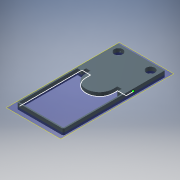
# Autodesk Inventor part: Cup_Dispenser_Slider
Saved by Autodesk Inventor 2016 (Build 200138000, 138)
## iProperties
Created: 2015-07-09
Part Number: Cup_Dispenser_Slider
Material: Generic
Document SubType Name: Modeling
Designer: marku
Density: 1 g/cm^3
Appearance: Lead
Author: marku
Autodesk Inventor part; units mm, degrees
ref_plane "YZ Plane" through (0, 0, 0) normal (1, 0, 0) x (0, 1, 0)
ref_plane "XZ Plane" through (0, 0, 0) normal (0, 1, 0) x (-1, 0, 0)
ref_plane "XY Plane" through (0, 0, 0) normal (0, 0, 1) x (1, 0, 0)
sketch "Sketch2" plane through (0, 0, 0) normal (0, 0, 1) x (1, 0, 0)
  line L0 (54, 117.2078) -> (54, -112.7922)
  arc A0 (50, -116.7922) -> (54, -112.7922) centre (50, -112.7922) ccw
  line L1 (50, -116.7922) -> (-50, -116.7922)
  arc A1 (-54, -112.7922) -> (-50, -116.7922) centre (-50, -112.7922) ccw
  line L2 (-54, -112.7922) -> (-54, 117.2078)
  line L3 (51, 117.2078) -> (51, -112.7922)
  arc A2 (50, -113.7922) -> (51, -112.7922) centre (50, -112.7922) ccw
  line L4 (50, -113.7922) -> (-50, -113.7922)
  arc A3 (-51, -112.7922) -> (-50, -113.7922) centre (-50, -112.7922) ccw
  line L5 (-51, -112.7922) -> (-51, 117.2078)
  line L6 (54, 117.2078) -> (-54, 117.2078)
  line L7 (-51, 114.2078) -> (51, 114.2078)
  dimension "d99" = 3
  dimension "d100" = 3
  constraints: 16 end point, 8 point on circle, 4 centre point, 2 horizontal, 2 point on line, 2 vertical, 1 perpendicular, 14 other
  measures "d99" distance between parallel lines of L0 L3
  measures "d100" distance between parallel lines of L6 L7
ref_plane "Work Plane1" through (-57, -119.7922, 15) normal (0, 0, -1) x (0, 1, 0)
ref_plane "Work Plane3" through (-57, -119.7922, 15) normal (0, 0, -1) x (0, 1, 0)
extrude "Extrusion1" add sketch "Sketch2" along normal up to surface (15 mm away) contours L0 A0 L1 A1 L2 L6 L5 A3 L4 A2 L3 | L3 L7 L5 L6
sketch "Sketch3" plane through (0, 0, 0) normal (0, 0, -1) x (-1, 0, 0)
  arc A0 (31.25, 57.2078) -> (-31.25, 57.2078) centre (0, 57.2078) ccw
  line L0 (-54, -112.7922) -> (-54, 114.2078) projected
  line L1 (-31.25, 57.2078) -> (-31.25, 47.2078)
  line L2 (-31.25, 47.2078) -> (-51, 47.2078)
  line L3 (31.25, 57.2078) -> (31.25, 47.2078)
  line L4 (31.25, 47.2078) -> (51, 47.2078)
  line L5 (-51, 114.2078) -> (51, 114.2078) projected
  line L6 (-51, -112.7922) -> (-51, 114.2078) projected
  line L7 (51, 114.2078) -> (51, -112.7922) projected
  circle A1 centre (0, 57.2078) radius 54 construction
  point P0 (0, 0)
  dimension "d8" = 31.25
  dimension "d9" = 10
  dimension "d10" = 10
  constraints: 8 end point, 4 point on line, 2 perpendicular, 2 point on circle, 1 centre point, 1 coincident, 1 tangent, 1 vertical
  measures "d8" radius of A0
  measures "d9" distance of L1.start L1.end
  measures "d10" distance of L3.start L3.end
extrude "Extrusion2" add sketch "Sketch3" against normal blind 3
ref_plane "Work Plane2" through (0, 0, 6) normal (0, 0, -1) x (-1, 0, 0)
sketch "Sketch4" plane through (0, 0, 6) normal (0, 0, -1) x (-1, 0, 0)
  line L0 (-31.25, 47.2078) -> (-51, 47.2078) construction
  circle A0 centre (0, 20.6666) radius 41 construction
  arc A1 (-31.25, 20.6666) -> (31.25, 20.6666) centre (0, 20.6666) ccw
  line L1 (-31.25, 20.6666) -> (-31.25, 30.6666)
  line L2 (31.25, 20.6666) -> (31.25, 30.6666)
  line L3 (31.25, 30.6666) -> (51, 30.6666)
  line L4 (-31.25, 30.6666) -> (-51, 30.6666)
  arc A2 (-51, -112.7922) -> (-50, -113.7922) centre (-50, -112.7922) ccw projected
  line L5 (-50, -113.7922) -> (50, -113.7922) projected
  arc A3 (50, -113.7922) -> (51, -112.7922) centre (50, -112.7922) ccw projected
  line L6 (51, -112.7922) -> (51, 114.2078) projected
  line L7 (51, 114.2078) -> (-51, 114.2078) projected
  line L8 (-51, 114.2078) -> (-51, -112.7922) projected
  arc A4 (-54, -112.7922) -> (-50, -116.7922) centre (-50, -112.7922) ccw projected
  line L9 (-54, -112.7922) -> (-54, 117.2078) projected
  line L10 (-54, 117.2078) -> (54, 117.2078) projected
  line L11 (54, 117.2078) -> (54, -112.7922) projected
  arc A5 (50, -116.7922) -> (54, -112.7922) centre (50, -112.7922) ccw projected
  line L12 (50, -116.7922) -> (-50, -116.7922) projected
  line L13 (0, 20.6666) -> (0, 0)
  dimension "d14" = 82
  dimension "d15" = 10
  dimension "d16" = 31.25
  constraints: 10 end point, 3 vertical, 2 perpendicular, 2 point on circle, 2 point on line, 2 tangent, 1 centre point, 1 coincident, 1 parallel, 3 other
  measures "d15" distance of L1.start L1.end
  measures "d16" radius of A1
extrude "Extrusion3" add sketch "Sketch4" against normal up to surface (9 mm away) contours L1 L4 L8 L7 L6 L3 L2 A1
sketch "Sketch5" plane through (0, 0, 3) normal (0, 0, 1) x (1, 0, 0)
  line L0 (-51, 47.2078) -> (-51, 114.2078) projected
  line L1 (-51, 47.2078) -> (-31.25, 47.2078) projected
  line L2 (-31.25, 47.2078) -> (-31.25, 57.2078) projected
  arc A0 (31.25, 57.2078) -> (-31.25, 57.2078) centre (0, 57.2078) ccw projected
  line L3 (31.25, 57.2078) -> (31.25, 47.2078) projected
  line L4 (31.25, 47.2078) -> (51, 47.2078) projected
  line L5 (51, 114.2078) -> (51, 47.2078) projected
  line L6 (-51, 114.2078) -> (51, 114.2078) projected
  line L7 (-41, 57.2078) -> (-41, 56.9578)
  line L8 (-41, 56.9578) -> (-41.25, 56.9578)
  line L9 (-41.25, 56.9578) -> (-41.25, 104.4578)
  line L10 (-41.25, 104.4578) -> (41.25, 104.4578)
  line L11 (41.25, 104.4578) -> (41.25, 56.9578)
  line L12 (41.25, 56.9578) -> (41, 56.9578)
  line L13 (41, 56.9578) -> (41, 57.2078)
  arc A1 (41, 57.2078) -> (-41, 57.2078) centre (0, 57.2078) ccw
  line L14 (41, 57.2078) -> (41.125, 47.2078)
  line L15 (31.25, 47.2078) -> (51, 47.2078) projected
  line L16 (-41.25, 56.9578) -> (-41.125, 47.2078)
  line L17 (-51, 47.2078) -> (-31.25, 47.2078) projected
  point P0 (0, 0)
  dimension "d101" = 41
  constraints: 18 end point, 2 midpoint, 2 point on circle, 1 centre point, 7 other
  measures "d101" distance of A0.centre L7.start
extrude "Extrusion4" add sketch "Sketch5" along normal up to surface (12 mm away) contours L0 L6 L5 L4 L14 L12 L11 L10 L9 L16 L1 | L9 L10 L11 L12 L14 A1 L7 L8
sketch "Sketch6" plane through (0, 0, 6) normal (0, 0, -1) x (-1, 0, 0)
  line L0 (-41.125, 47.2078) -> (-41, 57.2078) projected
  arc A0 (41, 57.2078) -> (-41, 57.2078) centre (0, 57.2078) ccw projected
  line L1 (41, 57.2078) -> (41, 56.9578) projected
  line L2 (41, 56.9578) -> (41.25, 56.9578) projected
  line L3 (41.25, 56.9578) -> (41.125, 47.2078) projected
  line L4 (41.125, 47.2078) -> (31.25, 47.2078) projected
  line L5 (31.25, 47.2078) -> (31.25, 57.2078) projected
  arc A1 (31.25, 57.2078) -> (-31.25, 57.2078) centre (0, 57.2078) ccw projected
  line L6 (-31.25, 57.2078) -> (-31.25, 47.2078) projected
  line L7 (-31.25, 47.2078) -> (-41.125, 47.2078) projected
  line L8 (-54, -112.7922) -> (-54, 117.2078) projected
  line L9 (-54, 117.2078) -> (54, 117.2078) projected
  line L10 (54, 117.2078) -> (54, -112.7922) projected
  arc A2 (50, -116.7922) -> (54, -112.7922) centre (50, -112.7922) ccw projected
  line L11 (50, -116.7922) -> (-50, -116.7922) projected
  arc A3 (-54, -112.7922) -> (-50, -116.7922) centre (-50, -112.7922) ccw projected
  line L12 (-31.25, 30.6666) -> (-51, 30.6666) projected
  line L13 (-31.25, 20.6666) -> (-31.25, 30.6666) projected
  arc A4 (-31.25, 20.6666) -> (31.25, 20.6666) centre (0, 20.6666) ccw projected
  line L14 (31.25, 30.6666) -> (31.25, 20.6666) projected
  line L15 (51, 30.6666) -> (31.25, 30.6666) projected
  line L16 (51, -112.7922) -> (51, 30.6666) projected
  line L17 (-51, 30.6666) -> (-51, -112.7922) projected
  line L18 (-51, 30.6666) -> (-31.25, 30.6666) projected
  line L19 (-41.125, 47.2078) -> (-51, 47.2078) projected
  line L20 (-41.125, 30.6666) -> (-41.125, 47.2078) construction
  line L21 (-41.125, 30.6666) -> (-41.125, 20.6666)
  arc A5 (-41.125, 20.6666) -> (41.125, 20.6666) centre (0, 20.6666) ccw
  line L22 (41.125, 20.6666) -> (41.125, 30.6666)
  line L23 (31.25, 30.6666) -> (51, 30.6666) projected
  arc A6 (-51, -112.7922) -> (-50, -113.7922) centre (-50, -112.7922) ccw projected
  line L24 (-50, -113.7922) -> (50, -113.7922) projected
  arc A7 (50, -113.7922) -> (51, -112.7922) centre (50, -112.7922) ccw projected
  line L25 (-31.25, 30.6666) -> (-31.25, 20.6666) construction
  line L26 (-31.25, 20.6666) -> (-41.125, 20.6666) construction
  constraints: 8 end point, 3 vertical, 2 midpoint, 2 point on circle, 1 centre point, 1 coincident, 1 perpendicular
extrude "Extrusion5" [suppressed]
sketch "Sketch7" plane through (0, 0, 0) normal (0, 0, -1) x (-1, 0, 0)
  line L0 (54, 20.9166) -> (41, 20.9166) projected
  line L1 (41, 20.9166) -> (54, 20.9166) projected
  line L2 (54, 56.9578) -> (41, 56.9578) projected
  line L3 (41, 56.9578) -> (54, 56.9578) projected
  line L4 (54, 47.2078) -> (54, 20.9166) projected
  line L5 (54, 56.9578) -> (54, 20.9166)
  line L6 (41, 56.9578) -> (41, 20.9166)
  line L7 (-41, 56.9578) -> (-54, 56.9578) projected
  line L8 (-41, 20.9166) -> (-54, 20.9166) projected
  line L9 (-41, 56.9578) -> (-41, 20.9166)
  line L10 (-54, 20.9166) -> (-54, 47.2078) projected
  line L11 (-54, 56.9578) -> (-54, 20.9166)
  point P0 (0, 0)
  constraints: 8 end point, 2 collinear, 2 vertical
extrude "Extrusion6" add sketch "Sketch7" against normal up to surface (15 mm away)
chamfer "Chamfer1" distance 6 distance2 3 1 edges at (36.125, 47.2078, 3) measured on face at (36.125, 47.7078, 3)
chamfer "Chamfer2" distance 6 distance2 3 1 edges at (-36.125, 47.2078, 3) measured on face at (-36.125, 47.7078, 3)
sketch "Sketch12" plane through (41, 30.6666, 15) normal (-1, 0, 0) x (0, 0, 1)
  line L0 (-15, 16.5412) -> (-12, 22.5412) construction
  line L1 (-12, 22.5412) -> (-3, 35.3946)
  line L2 (-0.6473, -143.4588) -> (-0.6473, 86.5412)
  line L3 (-3, 35.3946) -> (-3, 86.5412)
  line L4 (-15.6473, 86.5412) -> (-0.6473, 86.5412)
  line L5 (-12, 22.5412) -> (-12, 86.5412)
  line L6 (-12, 86.5412) -> (-3, 86.5412)
  point P0 (-15, -30.6666)
  point P1 (-12, 22.5412)
  dimension "d93" = 9
  dimension "d94" = 35
  constraints: 14 end point, 2 point on line, 2 vertical, 1 coincident, 1 collinear, 1 perpendicular
  measures "d93" horizontal distance of L0.end L1.end
  measures "d94" angle of L2 L1
extrude "Extrusion10" add sketch "Sketch12" along normal up to next
sketch "Sketch13" plane through (0, 57.2078, 12) normal (0, 0, 1) x (1, 0, 0)
  line L0 (31.25, 0) -> (31.25, -4) projected
  line L1 (-31.25, -4) -> (-31.25, 0) projected
  arc A0 (31.25, 0) -> (-31.25, 0) centre (0, 0) ccw projected
  line L2 (31.25, -4) -> (-31.25, -4) projected
  point P0 (0, -57.2078)
extrude "Extrusion11" [suppressed]
chamfer "Chamfer4" distance 0.75 angle 45 2 edges at (36.125, 30.6666, 6) (-36.125, 30.6666, 6)
sketch "Sketch8" plane through (-57, 117.2078, 15) normal (0, 0, 1) x (1, 0, 0)
  arc A0 (98, -60) -> (16, -60) centre (57, -60) ccw construction
  arc A1 (16, -96.5412) -> (98, -96.5412) centre (57, -96.5412) ccw construction
  line L0 (57, -60) -> (57, -96.5412) construction
  circle A2 centre (57, -180) radius 57 construction
  line L1 (57, -180) -> (142.4239, -180) construction
  line L2 (57, -161.7294) -> (57, -198.2706) construction
  circle A3 centre (57, -180) radius 18.2706 construction
  line L3 (38.7294, -198.2706) -> (75.2706, -198.2706) construction
  line L4 (38.7294, -201.2706) -> (75.2706, -201.2706)
  line L5 (75.2706, -195.2706) -> (38.7294, -195.2706)
  arc A4 (38.7294, -195.2706) -> (38.7294, -201.2706) centre (38.7294, -198.2706) ccw
  arc A5 (75.2706, -201.2706) -> (75.2706, -195.2706) centre (75.2706, -198.2706) ccw
  line L6 (75.2706, -180) -> (75.2706, -198.2706) construction
  point P0 (57, -117.2078)
  dimension "d33" = 6
  constraints: 16 end point, 6 point on circle, 6 tangent, 3 centre point, 2 horizontal, 2 midpoint, 2 vertical, 1 coincident, 1 collinear, 1 parallel, 1 perpendicular, 1 point on line, 1 symmetric about line
  measures "d33" diameter of A5
extrude "Extrusion7" cut sketch "Sketch8" against normal up to surface (15 mm away)
chamfer "Chamfer3" [suppressed]
sketch "Sketch10" plane through (-54, 117.2078, 15) normal (0, 1, 0) x (1, 0, 0)
  line L0 (0, 15) -> (0, 0) construction
  line L1 (108, 0) -> (0, 0) construction
  line L2 (108, 15) -> (108, 0) construction
  line L3 (0, 15) -> (108, 15) construction
  line L4 (108, 0) -> (0, 0) projected
  line L5 (54, 0) -> (54, 15) construction
  line L6 (108, 7.5) -> (0, 7.5) construction
  line L7 (0, 15) -> (0, 0) projected
  point P0 (96, 7.5)
  point P1 (12, 7.5)
  dimension "d102" = 12
  constraints: 4 end point, 4 midpoint, 2 point on line, 1 symmetric about line
  measures "d102" distance from line of L2 point (96, 7.5)
hole "Hole1" at (42, 117.2078, 7.5) at (-42, 117.2078, 7.5) direction (0, -1, 0) diameter 3 depth 8 tip angle 118
thicken "Thicken1" operation add thickness 0.8 both sides no extend neighbours yes toward (0, 0, -1) faces at (-10.4167, 88.3607, 15) (-1.2556, 107.5485, 0)
sketch "Sketch11" plane through (-56.2, 117.2078, 14.2) normal (0, 0, 1) x (1, 0, 0)
  circle A0 centre (56.2, -150.5412) radius 12
  line L0 (87.45, -86.5412) -> (97.2, -86.5412) construction
  line L1 (87.45, -96.5412) -> (87.45, -86.5412) construction
  arc A1 (24.95, -96.5412) -> (87.45, -96.5412) centre (56.2, -96.5412) ccw construction
  line L2 (24.95, -86.5412) -> (24.95, -96.5412) construction
  line L3 (15.2, -86.5412) -> (24.95, -86.5412) construction
  circle A2 centre (88.2, -150.5412) radius 12
  circle A3 centre (24.2, -150.5412) radius 12
  circle A4 centre (72.2, -178.2541) radius 12
  line L4 (56.2, -150.5412) -> (72.2, -178.2541) construction
  line L5 (72.2, -178.2541) -> (88.2, -150.5412) construction
  line L6 (88.2, -150.5412) -> (56.2, -150.5412) construction
  circle A5 centre (40.2, -178.2541) radius 12
  circle A6 centre (93.2, -198.2706) radius 10
  circle A7 centre (19.2, -198.2706) radius 10
  line L7 (56.2, -60) -> (56.2, -293.0623) construction
  circle A8 centre (72.2, -218.2706) radius 10
  line L8 (72.2, -178.2541) -> (72.2, -218.2706) construction
  circle A9 centre (40.2, -218.2706) radius 10
  circle A10 centre (19.2, -16) radius 10
  circle A11 centre (93.2, -16) radius 10
  line L9 (93.2, -16) -> (93.2, -198.2706) construction
  arc A12 (74.4706, -201.2706) -> (74.4706, -195.2706) centre (74.4706, -198.2706) ccw construction
  line L10 (93.2, -198.2706) -> (74.4706, -198.2706) construction
  line L11 (15.2, -96.2912) -> (15.2, -86.5412) projected
  line L12 (97.2, -86.5412) -> (97.2, -96.2912) projected
  line L13 (97.2, -96.2912) -> (107.2, -96.2912) projected
  line L14 (107.2, -96.2912) -> (107.2, -230) projected
  arc A13 (106.2, -231) -> (107.2, -230) centre (106.2, -230) ccw projected
  line L15 (106.2, -231) -> (6.2, -231) projected
  arc A14 (5.2, -230) -> (6.2, -231) centre (6.2, -230) ccw projected
  line L16 (5.2, -230) -> (5.2, -96.2912) projected
  line L17 (5.2, -96.2912) -> (15.2, -96.2912) projected
  point P0 (56.2, -117.2078)
  dimension "d56" = 24
  dimension "d59" = 32
  dimension "d66" = 32
  dimension "d71" = 24
  dimension "d74" = 32
  dimension "d79" = 20
  dimension "d80" = 20
  dimension "d81" = 20
  dimension "d82" = 20
  dimension "d83" = 5
  dimension "d85" = 54
  constraints: 14 end point, 11 centre point, 3 symmetric about line, 3 vertical, 2 equal length, 2 horizontal, 1 point on line, 2 other
  measures "d56" diameter of A0
  measures "d59" distance of L4.start L5.end
  measures "d66" distance of L4.start A3.centre
  measures "d71" diameter of A4
  measures "d74" distance of L4.end A5.centre
  measures "d79" diameter of A6
  measures "d80" diameter of A7
  measures "d81" diameter of A8
  measures "d82" diameter of A10
  measures "d83" distance from line of L5.end L9
  measures "d85" distance of A1.centre L4.start
extrude "Extrusion9" cut sketch "Sketch11" against normal up to surface (13.4 mm away)
equation "\"d99\" = thickness"
equation "\"d100\" = thickness"
equation "\"d8\" = cup_small_radius"
equation "\"d9\" = elongation"
equation "\"d10\" = d9"
equation "\"d11\" = thickness"
equation "\"d14\" = 2 * radius_tolerance + 2 * cup_big_radius"
equation "\"d15\" = elongation"
equation "\"d16\" = cup_small_radius"
equation "\"d17\" = thickness"
equation "\"d101\" = cup_big_radius + radius_tolerance"
equation "\"d20\" = thickness"
equation "\"d102\" = 4 * thickness"
equation "\"d23\" = thickness"
equation "\"d25\" = thickness"
equation "\"d27\" = 0.6 * elongation"
equation "\"d28\" = thickness"
equation "\"d30\" = 0.6 * elongation"
equation "\"d31\" = thickness"
equation "\"d93\" = 3 * thickness"
equation "\"d89\" = 0.25 * thickness"
equation "\"d90\" = thickness"
equation "\"d33\" = 2 * thickness"
equation "\"d34\" = thickness"
equation "\"d36\" = 0.5 * thickness"
equation "\"d37\" = thickness"
equation "\"d87\" = thickness"
equation "\"thickness\" = 3"
equation "\"cup_to_cup_distance\" = 4"
equation "\"cup_lid_end_height\" = 2"
equation "\"cup_gap\" = 2"
equation "\"cup_lid_height\" = 5"
equation "\"cup_small_radius\" = 31.25"
equation "\"cup_big_radius\" = 39"
equation "\"elongation\" = 10"
equation "\"d13\" = -0.5 * cup_gap - cup_lid_height"
equation "\"radius_tolerance\" = 2"
equation "\"bearing_tolerance\" = 1"
body "Solid1"
